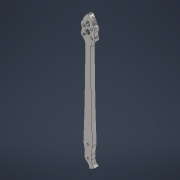
# Autodesk Inventor part: 10inchfrontarm
Saved by Autodesk Inventor 2021 (Build 250183000, 183)
## iProperties
Created: 2020-05-02
Part Number: 10inchfrontarm
Material: Generic
Document SubType Name: Modeling
Designer: Logan
Density: 1 g/cm^3
Appearance: Diamond Plate
Mass: 17.3564 g
Surface Area: 89.1298 cm^2
Volume: 17.3564 cm^3
Author: Logan
Autodesk Inventor part; units mm, degrees
ref_plane "YZ Plane" through (0, 0, 0) normal (1, 0, 0) x (0, 1, 0)
ref_plane "XZ Plane" through (0, 0, 0) normal (0, 1, 0) x (-1, 0, 0)
ref_plane "XY Plane" through (0, 0, 0) normal (0, 0, 1) x (1, 0, 0)
sketch "Sketch1" plane through (0, 0, 0) normal (0, 0, 1) x (1, 0, 0)
  line L0 (0, 0) -> (0, 20) construction
  line L1 (0, 20) -> (0, 180) construction
  line L2 (4.5, 20) -> (4.5, 180)
  line L3 (-4.5, 180) -> (-4.5, 20)
  arc A0 (-4.5, 20) -> (4.5, 20) centre (0, 20) ccw
  arc A1 (4.5, 180) -> (-4.5, 180) centre (0, 180) ccw
  line L4 (-6.7175, 186.7175) -> (6.7175, 173.2825) construction
  line L5 (-10.253, 183.182) -> (3.182, 169.747)
  line L6 (10.253, 176.818) -> (-3.182, 190.253)
  arc A2 (-3.182, 190.253) -> (-10.253, 183.182) centre (-6.7175, 186.7175) ccw
  arc A3 (3.182, 169.747) -> (10.253, 176.818) centre (6.7175, 173.2825) ccw
  line L7 (0, 180) -> (19, 180) construction
  line L8 (-6.7175, 173.2825) -> (6.7175, 186.7175) construction
  line L9 (-3.182, 169.747) -> (10.253, 183.182)
  line L10 (3.182, 190.253) -> (-10.253, 176.818)
  arc A4 (-10.253, 176.818) -> (-3.182, 169.747) centre (-6.7175, 173.2825) ccw
  arc A5 (10.253, 183.182) -> (3.182, 190.253) centre (6.7175, 186.7175) ccw
  line L11 (0, 180) -> (19, 180) construction
  line L12 (0, 180) -> (0, 202)
  arc A6 (6.7175, 186.7175) -> (0, 202) centre (-18.2146, 184.8761) ccw construction
  arc A7 (9.7094, 186.9385) -> (2.1857, 204.0549) centre (-18.2146, 184.8761) ccw
  arc A8 (3.7257, 186.4965) -> (-2.1857, 199.9451) centre (-18.2146, 184.8761) ccw
  arc A9 (3.7257, 186.4965) -> (9.7094, 186.9385) centre (6.7175, 186.7175) ccw
  arc A10 (2.1857, 204.0549) -> (-2.1857, 199.9451) centre (0, 202) ccw
  arc A11 (0, 202) -> (-6.7175, 186.7175) centre (18.2146, 184.8761) ccw construction
  arc A12 (-2.1857, 204.0549) -> (-9.7094, 186.9385) centre (18.2146, 184.8761) ccw
  arc A13 (2.1857, 199.9451) -> (-3.7257, 186.4965) centre (18.2146, 184.8761) ccw
  arc A14 (2.1857, 199.9451) -> (-2.1857, 204.0549) centre (0, 202) ccw
  arc A15 (-9.7094, 186.9385) -> (-3.7257, 186.4965) centre (-6.7175, 186.7175) ccw
  circle A16 centre (-6.7175, 186.7175) radius 1.5
  circle A17 centre (6.7175, 186.7175) radius 1.5
  circle A18 centre (6.7175, 173.2825) radius 1.5
  circle A19 centre (-6.7175, 173.2825) radius 1.5
  circle A20 centre (0, 180) radius 3.5
  circle A21 centre (0, 20) radius 1.5
  circle A22 centre (0, 0) radius 1.5
  circle A23 centre (0, 20) radius 7.5
  line L13 (0, 20) -> (0, 0) construction
  line L14 (-5.5, 20) -> (-5.5, 0)
  line L15 (5.5, 0) -> (5.5, 20)
  arc A24 (5.5, 20) -> (-5.5, 20) centre (0, 20) ccw
  arc A25 (-5.5, 0) -> (5.5, 0) centre (0, 0) ccw
  line L16 (0, 0) -> (13.5, -23.3827)
  line L17 (0, 0) -> (27, 0) construction
  line L18 (6.75, -11.6913) -> (11.0801, -9.1913)
  line L19 (6.75, -11.6913) -> (11.75, -11.6913) construction
  line L20 (6.75, -11.6913) -> (2.4199, -14.1913)
  line L21 (6.75, -11.6913) -> (11.75, -11.6913) construction
  line L22 (0, 0) -> (4.3301, 2.5)
  line L23 (0, 0) -> (5, 0) construction
  line L24 (0, 0) -> (-4.3301, -2.5)
  line L25 (0, 0) -> (5, 0) construction
  arc A26 (2.4199, -14.1913) -> (-4.3301, -2.5) centre (-9.5475, -13.3065) ccw
  arc A27 (4.3301, 2.5) -> (11.0801, -9.1913) centre (16.2975, 1.6151) ccw
  circle A28 centre (-5.6569, 185.6569) radius 1.5
  circle A29 centre (5.6569, 185.6569) radius 1.5
  circle A30 centre (5.6569, 174.3431) radius 1.5
  circle A31 centre (-5.6569, 174.3431) radius 1.5
  point P0 (0, 10)
  point P1 (0, 100)
  point P2 (-7.0711, 180)
  point P3 (-4.5, 168.8011)
  point P4 (4.5, 168.8011)
  point P5 (7.0711, 180)
  point P6 (9.0793, 191.1245)
  point P7 (-2.1857, 204.0549)
  point P8 (-9.0793, 191.1245)
  point P9 (0, 187.0711)
  point P10 (-3.131, 190.2021)
  point P11 (0, 197.2142)
  point P12 (3.131, 190.2021)
  point P13 (0, 10)
  point P14 (-4.5, 26)
  point P15 (-5.5, 14.901)
  point P16 (5.5, 14.901)
  point P17 (4.5, 26)
  point P18 (4.972, -2.3515)
  point P19 (-0.4496, -5.4816)
  point P20 (5.2686, 187.1057)
  point P21 (7.1057, 185.2686)
  point P22 (-7.1057, 185.2686)
  point P23 (-5.2686, 187.1057)
  point P24 (7.1057, 174.7314)
  point P25 (5.2686, 172.8943)
  point P26 (-5.2686, 172.8943)
  point P27 (-7.1057, 174.7314)
  dimension "d15" = 3
  dimension "d16" = 3
  dimension "d17" = 3
  dimension "d18" = 3
  dimension "d0" = 20
  dimension "d2" = 160
  dimension "d3" = 9
  dimension "d4" = 9.5
  dimension "d5" = 45
  dimension "d6" = 10
  dimension "d7" = 9.5
  dimension "d8" = 45
  dimension "d9" = 10
  dimension "d10" = 22
  dimension "d11" = 25
  dimension "d12" = 6
  dimension "d13" = 25
  dimension "d14" = 6
  dimension "d19" = 7
  dimension "d20" = 3
  dimension "d21" = 3
  dimension "d27" = 15
  dimension "d28" = 11
  dimension "d29" = 27
  dimension "d30" = 60
  dimension "d31" = 5
  dimension "d32" = 30
  dimension "d33" = 5
  dimension "d34" = 150
  dimension "d35" = 5
  dimension "d36" = 30
  dimension "d37" = 5
  dimension "d38" = 150
  dimension "d39" = 12
  dimension "d40" = 12
  dimension "d41" = 3
  dimension "d42" = 3
  dimension "d43" = 3
  dimension "d44" = 3
  constraints: 62 end point, 40 point on circle, 28 centre point, 24 tangent, 8 coincident, 7 equal length, 7 horizontal, 6 midpoint, 5 point on line, 4 parallel, 3 vertical, 1 perpendicular, 12 other
  measures "d0" distance of L0.start L0.end
  measures "d2" distance of L0.end L1.end
  measures "d3" diameter of A1
  measures "d4" distance of L1.end L4.end
  measures "d5" angle of L4 L7
  measures "d6" diameter of A3
  measures "d7" distance of L1.end L8.end
  measures "d8" angle of L11 L8
  measures "d9" diameter of A5
  measures "d10" distance of L1.end L12.end
  measures "d11" radius of A6
  measures "d12" diameter of A9
  measures "d13" radius of A11
  measures "d14" diameter of A15
  measures "d19" diameter of A20
  measures "d20" diameter of A21
  measures "d21" diameter of A22
  measures "d27" diameter of A23
  measures "d28" diameter of A25
  measures "d29" distance of L13.end L16.end
  measures "d30" angle of L16 L17
  measures "d31" distance of L18.start L18.end
  measures "d32" angle of L19 L18
  measures "d33" distance of L18.start L20.end
  measures "d34" angle of L20 L21
  measures "d35" distance of L13.end L22.end
  measures "d36" angle of L23 L22
  measures "d37" distance of L13.end L24.end
  measures "d38" angle of L24 L25
  measures "d39" radius of A26
  measures "d40" radius of A27
  measures "d41" diameter of A28
  measures "d42" diameter of A29
  measures "d43" diameter of A30
  measures "d44" diameter of A31
extrude "Extrusion1" add sketch "Sketch1" along normal blind 7 contours A0 L3 A24 L2 | L2 A24 L15 A23 L14 L3 A0 | A24 L3 A23 L2 | L2 A23 L15 A24 | A23 L3 A4 L9 L5 A3 L2 | A24 L14 A23 L3 | A3 L5 L9 L2 A30 | L2 A30 A18 L9 L6 A3 | L15 A25 A27 L22 A22 L24 A26 L14 A23 | A4 L10 L5 L3 A31 A19 | L3 A31 L5 L9 A4 | L5 L3 A1 L2 L9 | L9 L2 A1 L12 L6 | L6 L10 A8 A9 A7 A5 L9 | A27 L18 L16 A25 | A25 L16 A22 L22 A27 | L5 L10 L12 A1 L3 | L10 L5 A2 A12 A15 A13 L6 | A26 L24 A22 L16 A25 | A25 L16 L20 A26 | A13 A15 A12 A2 L6 | L6 A2 A12 A10 A8 A13 | A8 A13 A14 A7 A5 L10 | L10 A5 A7 A9 A8 | A8 A10 A14 A13
fillet "Fillet1" radius 3500 2 edges at (4.5, 26, 3.5) (-4.5, 26, 3.5)
fillet "Fillet2" radius 10 8 edges at (-9.0793, 191.1245, 3.5) (-7.0711, 180, 3.5) (-4.5, 168.8011, 3.5) (4.5, 168.8011, 3.5) (7.0711, 180, 3.5) (9.0793, 191.1245, 3.5) (4.972, -2.3515, 3.5) (-0.4496, -5.4816, 3.5)
fillet "Fillet3" radius 1.6 4 edges at (0, 197.2142, 3.5) (-3.131, 190.2021, 3.5) (0, 187.0711, 3.5) (3.131, 190.2021, 3.5)
fillet "Fillet4" radius 40 2 edges at (-5.5, 14.901, 3.5) (5.5, 14.901, 3.5)
body "Solid1"
